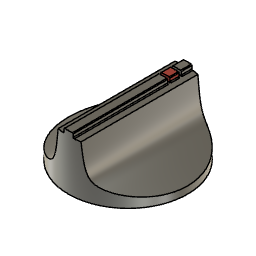
dial X1 v5 (Autodesk Fusion 360 design; units mm, degrees)
Autodesk Fusion 360 part; units mm, degrees
note: some values were not read from the file. Chosen so that the rebuilt part matches the saved one: that a step has no effect. Set by a fixed rule: which sketch regions a step uses.
sketch "Main Cylinder" plane through (0, 0, 0) normal (0, 0, 1) x (1, 0, 0)
  circle A0 centre (0, 0) radius 20.75
  dimension "d1" = 41.5
  constraint coincident A0.centre origin
  measures "d1" diameter of A0
extrude "Extrude1" add sketch "Main Cylinder" along normal blind 3.2 makes body 1
delete_body "RemoveBody1" bodies 1
extrude "Extrude2" add sketch "Main Cylinder" along normal blind 19.4 separate body makes body 2
sketch "cross-section" plane through (0, 0, 0) normal (0, 1, 0) x (1, 0, 0)
  circle A0 through (-20.75, 0, 0) (10.375, 0, 17.97) (10.375, 0, -17.97)
  line L0 (0, 0) -> (20.75, 0)
  line L1 (20.75, 0) -> (20.75, -2.5)
  spline S0 degree 2 poles (20.75, -2.5) (5.3, -5.3) (4, -17.6) knots 0 0 0 2.577894 2.577894 2.577894 weights 1 3 1
  line L2 (4, -17.6) -> (1.9, -17.6)
  line L3 (1.6, -17.9) -> (1.6, -18.95)
  line L4 (1.35, -19.2) -> (0, -19.2)
  line L5 (0, -19.2) -> (0, 0)
  line L6 (0, 0) -> (6.7175, -6.7175) construction
  line L7 (0, 0) -> (11, 0) construction
  line L8 (0, 0) -> (0, -28) construction
  line L9 (-20.75, 0) -> (-20.75, -2.5)
  spline S1 degree 2 poles (-20.75, -2.5) (-5.3, -5.3) (-4, -17.6) knots 0 0 0 2.577894 2.577894 2.577894 weights 1 3 1
  line L10 (-4, -17.6) -> (-1.9, -17.6)
  line L11 (-1.6, -17.9) -> (-1.6, -18.95)
  line L12 (-1.35, -19.2) -> (0, -19.2)
  line L13 (0, -19.2) -> (0, 0)
  line L14 (0, 0) -> (-20.75, 0)
  arc A1 (-1.6, -18.95) -> (-1.35, -19.2) centre (-1.35, -18.95) ccw
  arc A2 (1.35, -19.2) -> (1.6, -18.95) centre (1.35, -18.95) ccw
  arc A3 (1.9, -17.6) -> (1.6, -17.9) centre (1.9, -17.9) ccw
  arc A4 (-1.6, -17.9) -> (-1.9, -17.6) centre (-1.9, -17.9) ccw
  dimension "d10" = 4
  dimension "d11" = 45
  dimension "d12" = 9.5
  dimension "d13" = 19.2
  dimension "d38" = 2.5
  dimension "d39" = 0.25
  dimension "d40" = 1.6
  dimension "d41" = 0.3
  dimension "d42" = 0.3
  constraint coincident L0.start L5.end
  constraint horizontal L0
  constraint perpendicular L0 L1
  constraint horizontal L2
  constraint perpendicular L2 L3
  constraint perpendicular L3 L4
  constraint vertical L5
  constraint horizontal L4
  constraint vertical L1
  constraint vertical L3
  constraint horizontal L7
  constraint perpendicular L7 L8
  constraint symmetric L0.start L8 L5.end
  constraint symmetric L0.end L8 L9.start
  constraint symmetric L1.end L8 L9.end
  constraint symmetric S0.end L8 S1.end
  constraint symmetric S0 L8 S1
  constraint symmetric L4.end L8 L5.start
  constraint tangent L12 A1
  constraint tangent L11 A1
  constraint symmetric L8 L12.start L4.start
  constraint symmetric L8 L11.end L3.end
  constraint symmetric L8 A1 A2
  constraint tangent L3 A3
  constraint tangent L2 A3
  constraint tangent L10 A4
  constraint tangent L11 A4
  measures "d10" distance of S0.end L5
  measures "d11" angle of L6 L7
  measures "d12" distance of L0.start L6.end
  measures "d13" distance of L4.end L0.start
  measures "d38" distance of L9.start L9.end
  measures "d39" radius of A1
  measures "d40" distance of L3 L5
  measures "d41" radius of A3
  measures "d42" radius of A4
extrude "Extrude4" [no effect]
extrude "Extrude5" cut sketch "cross-section" along normal mid plane 42 keep common part bodies 2
extrude "Extrude6" cut sketch "cross-section" along normal mid plane 44 keep common part bodies 2
sketch "top cuts" plane through (0, 0, 19.2) normal (0, 0, 1) x (-1, 0, 0)
  arc A0 (1.35, 20.706) -> (-1.35, 20.706) centre (0, 0) ccw
  line L0 (2.5365, -16.9923) -> (-2.7233, -16.9923)
  line L1 (-2.7233, -16.9923) -> (-2.7233, -16.1923)
  line L2 (-2.7233, -16.1923) -> (2.5365, -16.1923)
  line L3 (2.5365, -16.1923) -> (2.5365, -16.9923)
  line L4 (2.5365, -12.9923) -> (-2.7233, -12.9923)
  line L5 (-2.7233, -12.9923) -> (-2.7233, -12.1923)
  line L6 (-2.7233, -12.1923) -> (2.5365, -12.1923)
  line L7 (2.5365, -12.1923) -> (2.5365, -12.9923)
  line L8 (-1.35, 20.706) -> (-1.35, -20.706)
  arc A1 (-1.35, -20.706) -> (1.35, -20.706) centre (0, 0) ccw
  line L9 (1.35, -20.706) -> (1.35, 20.706)
  dimension "d23" = 0.8
  dimension "d25" = 3.2
  constraint horizontal L0
  constraint vertical L1
  constraint horizontal L2
  constraint vertical L3
  constraint horizontal L4
  constraint vertical L5
  constraint horizontal L6
  constraint vertical L7
  constraint equal L3 L7
  measures "d23" distance of L0.start L2.end
  measures "d25" distance of L2 L4
extrude "Extrude7" cut sketch "top cuts" against normal blind 1.6 contours L4 L6 L8 L9 | L4 L6 L7 L9 | L4 L5 L6 L8 | L0 L2 L8 L9 | L0 L2 L3 L9 | L0 L1 L2 L8 bodies 2
hole "Hole1" at (0.0943, -0.0053, 0) direction (0, 0, 1) diameter 6.5 depth 12 tip angle 180 countersink diameter 9 countersink angle 110 bodies 2
sketch "notches" plane through (0, 0, 0) normal (0, 0, 1) x (1, 0, 0)
  circle A0 centre (0, 3.15) radius 1
  line L0 (7.3845, 0) -> (-9.5008, 0) construction
  circle A1 centre (0, -3.15) radius 1
  line L1 (1.3336, -2.15) -> (-11.8392, -2.15) construction
  line L2 (1.3336, 2.15) -> (-11.8392, 2.15) construction
  line L3 (0, -5.037) -> (0, 5.037) construction
  dimension "d33" = 2
  dimension "d34" = 4.3
  constraint horizontal L0
  constraint symmetric A0 L0 A1
  constraint horizontal L1
  constraint tangent A1 L1
  constraint symmetric L0 L1.start L2.start
  constraint symmetric L0 L1.end L2.end
  constraint coincident origin L0
  constraint vertical L3
  constraint coincident origin L3
  constraint midpoint origin L3
  constraint coincident A1.centre L3
  measures "d33" diameter of A0
  measures "d34" distance of L1 L2
extrude "Extrude8" add sketch "notches" along normal blind 7 from surface at 1 bodies 2
sketch "Sketch6" plane through (0, 0, 0) normal (0, 0, -1) x (1, 0, 0)
  circle A0 centre (0.0943, 0.0053) radius 4.5
  circle A1 centre (0, 0) radius 20.75
